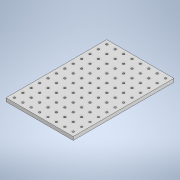
# Autodesk Inventor part: Optical Breadboard
Saved by Autodesk Inventor 2020 (Build 240168000, 168)
## iProperties
Created: 2024-01-28
Part Number: Optical Breadboard
Material: Generic
Document SubType Name: Modeling
Designer: Scott
Density: 1 g/cm^3
Appearance: Default
Author: Scott
Autodesk Inventor part; units mm, degrees
ref_plane "YZ Plane" through (0, 0, 0) normal (1, 0, 0) x (0, 1, 0)
ref_plane "XZ Plane" through (0, 0, 0) normal (0, 1, 0) x (-1, 0, 0)
ref_plane "XY Plane" through (0, 0, 0) normal (0, 0, 1) x (1, 0, 0)
sketch "Sketch1" plane through (0, 0, 0) normal (0, 0, 1) x (1, 0, 0)
  line L0 (0, 0) -> (200, 0)
  line L1 (200, 0) -> (200, -10)
  line L2 (200, -10) -> (0, -10)
  line L3 (0, -10) -> (0, 0)
  dimension "d0" = 200
  dimension "d1" = 10
  constraints: 8 end point, 3 perpendicular, 1 horizontal
  measures "d0" distance of L0.start L0.end
  measures "d1" distance of L0.end L1.end
extrude "Extrusion1" add sketch "Sketch1" along normal blind 300
sketch "Sketch2" plane through (0, 0, 0) normal (0, 1, 0) x (1, 0, 0)
  line L0 (0, 0) -> (0, -300) projected
  line L1 (0, 0) -> (0, -12.5)
  line L2 (0, -12.5) -> (12.5, -12.5)
  circle A0 centre (12.5, -12.5) radius 3
  dimension "d4" = 12.5
  dimension "d5" = 12.5
  dimension "d6" = 6
  constraints: 4 end point, 1 centre point, 1 coincident, 1 perpendicular, 1 point on line
  measures "d4" distance of L0.start L1.end
  measures "d5" distance of L1.end L2.end
  measures "d6" diameter of A0
extrude "Extrusion2" cut sketch "Sketch2" against normal blind 20
pattern_linear "Rectangular Pattern1" count 8 spacing 25 along (1, 0, 0) count 12 spacing 25 along (0, 0, 1) of "Extrusion2"
body "Solid1"
